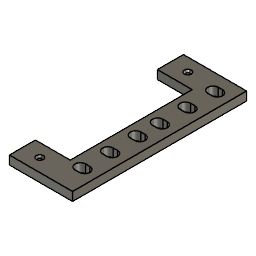
Main (Autodesk Fusion 360 archive; units mm, degrees)
design "Endcaps Right"
Autodesk Fusion 360 part; units mm, degrees
sketch "Sketch1" plane through (0, 0, 0) normal (0, 0, 1) x (1, 0, 0)
  line L0 (0, 0) -> (16.3, 0)
  line L1 (16.3, 0) -> (16.3, 100)
  line L2 (16.3, 100) -> (0, 100)
  line L3 (0, 100) -> (0, 0)
  line L4 (16.3, 100) -> (36.3, 100)
  line L5 (36.3, 100) -> (36.3, 85)
  line L6 (36.3, 85) -> (16.3, 85)
  line L7 (16.3, 85) -> (16.3, 100)
  line L8 (16.3, 0) -> (36.3, 0)
  line L9 (36.3, 0) -> (36.3, 15)
  line L10 (36.3, 15) -> (16.3, 15)
  line L11 (16.3, 15) -> (16.3, 0)
  line L12 (7.5, 87.65) -> (10, 87.65)
  arc A0 (10, 87.65) -> (10, 93.65) centre (10, 90.65) ccw
  line L13 (10, 93.65) -> (7.5, 93.65)
  arc A1 (7.5, 93.65) -> (7.5, 87.65) centre (7.5, 90.65) ccw
  line L14 (7.5, 90.65) -> (10, 90.65) construction
  arc A2 (10, 71.775) -> (10, 77.775) centre (10, 74.775) ccw
  line L15 (7.5, 71.775) -> (10, 71.775)
  arc A3 (7.5, 77.775) -> (7.5, 71.775) centre (7.5, 74.775) ccw
  line L16 (10, 77.775) -> (7.5, 77.775)
  arc A4 (10, 55.9) -> (10, 61.9) centre (10, 58.9) ccw
  line L17 (7.5, 55.9) -> (10, 55.9)
  arc A5 (7.5, 61.9) -> (7.5, 55.9) centre (7.5, 58.9) ccw
  line L18 (10, 61.9) -> (7.5, 61.9)
  line L19 (7.5, 43.2) -> (10, 43.2)
  arc A6 (7.5, 49.2) -> (7.5, 43.2) centre (7.5, 46.2) ccw
  line L20 (10, 49.2) -> (7.5, 49.2)
  arc A7 (10, 43.2) -> (10, 49.2) centre (10, 46.2) ccw
  line L21 (7.5, 27.325) -> (10, 27.325)
  arc A8 (7.5, 33.325) -> (7.5, 27.325) centre (7.5, 30.325) ccw
  line L22 (10, 33.325) -> (7.5, 33.325)
  arc A9 (10, 27.325) -> (10, 33.325) centre (10, 30.325) ccw
  line L23 (7.5, 11.45) -> (10, 11.45)
  arc A10 (7.5, 17.45) -> (7.5, 11.45) centre (7.5, 14.45) ccw
  line L24 (10, 17.45) -> (7.5, 17.45)
  arc A11 (10, 11.45) -> (10, 17.45) centre (10, 14.45) ccw
  circle A12 centre (26.3, 7.5) radius 1
  circle A13 centre (26.3, 92.5) radius 1
  point P0 (8.75, 90.65)
  dimension "d1" = 16.3
  dimension "d2" = 100
  dimension "d3" = 20
  dimension "d4" = 15
  dimension "d5" = 20
  dimension "d19" = 6
  dimension "d20" = 6
  dimension "d21" = 6
  dimension "d22" = 15.875
  dimension "d23" = 15.875
  dimension "d24" = 6
  dimension "d25" = 6
  dimension "d26" = 15.875
  dimension "d27" = 12.7
  dimension "d28" = 6
  dimension "d29" = 15.875
  dimension "d30" = 6.35
  dimension "d33" = 2
  dimension "d34" = 2
  constraint horizontal L0
  constraint vertical L1
  constraint horizontal L2
  constraint vertical L3
  constraint coincident L0.start L3.end
  constraint horizontal L4
  constraint vertical L5
  constraint horizontal L6
  constraint vertical L7
  constraint horizontal L8
  constraint vertical L9
  constraint horizontal L10
  constraint vertical L11
  constraint tangent L12 A0
  constraint tangent A0 L13
  constraint parallel L12 L13
  constraint tangent L13 A1
  constraint tangent L12 A1
  constraint horizontal L14
  constraint midpoint L14 P0
  constraint tangent A2 L15
  constraint tangent A2 L16
  constraint parallel L15 L16
  constraint tangent A3 L16
  constraint tangent L15 A3
  constraint tangent A4 L17
  constraint tangent A4 L18
  constraint parallel L17 L18
  constraint tangent A5 L18
  constraint tangent L17 A5
  constraint tangent L19 A7
  constraint tangent L20 A7
  constraint parallel L19 L20
  constraint tangent A6 L20
  constraint tangent L19 A6
  constraint tangent L21 A9
  constraint tangent L22 A9
  constraint parallel L21 L22
  constraint tangent A8 L22
  constraint tangent L21 A8
  constraint tangent L23 A11
  constraint tangent L24 A11
  constraint parallel L23 L24
  constraint tangent A10 L24
  constraint tangent L23 A10
  measures "d1" distance of L0.start L0.end
  measures "d2" distance of L0.start L2.end
  measures "d3" distance of L1.end L4.end
  measures "d4" distance of L1.end L6.end
  measures "d5" distance of L0.end L8.end
  measures "d19" diameter of A0
  measures "d20" diameter of A2
  measures "d21" diameter of A4
  measures "d22" distance of L13 L16
  measures "d23" distance of L16 L18
  measures "d24" diameter of A7
  measures "d25" diameter of A9
  measures "d26" distance of L20 L22
  measures "d27" distance of L18 L20
  measures "d28" diameter of A11
  measures "d29" distance of L22 L24
  measures "d30" distance of L2 L13
  measures "d33" diameter of A12
  measures "d34" diameter of A13
extrude "Extrude1" add sketch "Sketch1" along normal blind 5
sketch "Sketch2" plane through (0, 0, 5) normal (0, 0, 1) x (-1, 0, 0)
  arc A0 (-10, -11.45) -> (-10, -17.45) centre (-10, -14.45) ccw
  line L0 (-10, -11.45) -> (-7.5, -11.45)
  arc A1 (-7.5, -17.45) -> (-7.5, -11.45) centre (-7.5, -14.45) ccw
  line L1 (-7.5, -17.45) -> (-10, -17.45)
  line L2 (-7.5, -61.9) -> (-10, -61.9)
  arc A2 (-10, -55.9) -> (-10, -61.9) centre (-10, -58.9) ccw
  line L3 (-10, -55.9) -> (-7.5, -55.9)
  arc A3 (-7.5, -61.9) -> (-7.5, -55.9) centre (-7.5, -58.9) ccw
  arc A4 (-7.5, -93.65) -> (-7.5, -87.65) centre (-7.5, -90.65) ccw
  line L4 (-7.5, -93.65) -> (-10, -93.65)
  arc A5 (-10, -87.65) -> (-10, -93.65) centre (-10, -90.65) ccw
  line L5 (-10, -87.65) -> (-7.5, -87.65)
  line L6 (-7.5, -77.775) -> (-10, -77.775)
  arc A6 (-10, -71.775) -> (-10, -77.775) centre (-10, -74.775) ccw
  line L7 (-10, -71.775) -> (-7.5, -71.775)
  arc A7 (-7.5, -77.775) -> (-7.5, -71.775) centre (-7.5, -74.775) ccw
  arc A8 (-10, -43.2) -> (-10, -49.2) centre (-10, -46.2) ccw
  line L8 (-10, -43.2) -> (-7.5, -43.2)
  arc A9 (-7.5, -49.2) -> (-7.5, -43.2) centre (-7.5, -46.2) ccw
  line L9 (-7.5, -49.2) -> (-10, -49.2)
  circle A10 centre (-26.3, -7.5) radius 1
  arc A11 (-10, -27.325) -> (-10, -33.325) centre (-10, -30.325) ccw
  line L10 (-10, -27.325) -> (-7.5, -27.325)
  arc A12 (-7.5, -33.325) -> (-7.5, -27.325) centre (-7.5, -30.325) ccw
  line L11 (-7.5, -33.325) -> (-10, -33.325)
  circle A13 centre (-26.3, -92.5) radius 1
  line L12 (-36.3, -100) -> (0, -100)
  line L13 (0, -100) -> (0, 0)
  line L14 (0, 0) -> (-36.3, 0)
  line L15 (-36.3, 0) -> (-36.3, -15)
  line L16 (-36.3, -15) -> (-16.3, -15)
  line L17 (-16.3, -15) -> (-16.3, -85)
  line L18 (-16.3, -85) -> (-36.3, -85)
  line L19 (-36.3, -85) -> (-36.3, -100)
  circle A14 centre (-26.3, -7.5) radius 2
  circle A15 centre (-26.3, -92.5) radius 2
  dimension "d35" = 4
  dimension "d36" = 4
  constraint concentric A10 A14
  constraint concentric A13 A15
  measures "d35" diameter of A14
  measures "d36" diameter of A15
extrude "Extrude2" cut sketch "Sketch2" along normal blind 4.5 draft -45 from surface at -5 contours A10 | A13 | A14 | A15
move_body "Move1" bodies 1 to x (-1, 0, 0) y (0, 1, 0) z (0, 0, -1) at (36.7067, 0, 10)
move_body "Move2" bodies 1 to x (1, 0, 0) y (0, 1, 0) z (0, 0, 1) at (-0.4067, 0, -5)

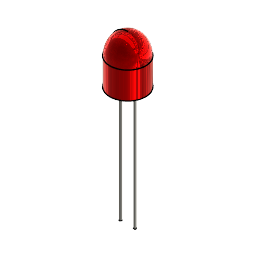
design "LED"
Autodesk Fusion 360 part; units mm, degrees
sketch "Sketch1" plane through (0, 0, 0) normal (0, 0, 1) x (1, 0, 0)
  circle A0 centre (0, 0) radius 1.5
  constraint coincident A0.centre origin
extrude "Extrude1" add sketch "Sketch1" along normal blind 4
fillet "Fillet1" offset 1.49 second offset 1.75 1 edges at (-1.3985, -0.5424, 4) measured on face at (-0.4452, -0.0508, 4)
sketch "Sketch2" plane through (0, 0, 0) normal (0, 0, -1) x (1, 0, 0)
  circle A0 centre (0, 0) radius 1.5
  circle A1 centre (0.6, 0) radius 0.1
  circle A2 centre (-0.6, 0) radius 0.1
extrude "Extrude2" add sketch "Sketch2" along normal blind 10 contours A1 | A2

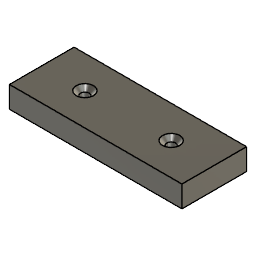
design "Cpnnector"
Autodesk Fusion 360 part; units mm, degrees
sketch "Sketch1" plane through (0, 0, 0) normal (0, 0, 1) x (1, 0, 0)
  line L0 (0, 0) -> (40, 0)
  line L1 (40, 0) -> (40, 15)
  line L2 (40, 15) -> (0, 15)
  line L3 (0, 15) -> (0, 0)
  circle A0 centre (10, 7.5) radius 1
  circle A1 centre (30, 7.5) radius 1
  circle A2 centre (30, 7.5) radius 2
  circle A3 centre (10, 7.5) radius 2
  constraint horizontal L0
  constraint vertical L1
  constraint horizontal L2
  constraint vertical L3
  constraint coincident L0.start L3.end
  constraint concentric A1 A2
  constraint concentric A0 A3
extrude "Extrude1" add sketch "Sketch1" along normal blind 5 contours L0 L1 L2 L3 | A2 | A3
extrude "Extrude2" cut sketch "Sketch1" against normal blind 1 draft -45 from surface at 5 contours A0 | A1 | A2 | A3

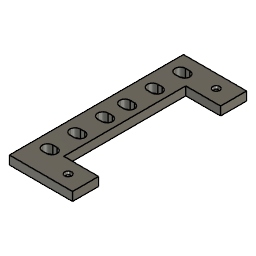
design "Endcaps Left"
Autodesk Fusion 360 part; units mm, degrees
sketch "Sketch1" plane through (0, 0, 0) normal (0, 0, 1) x (1, 0, 0)
  line L0 (0, 0) -> (16.3, 0)
  line L1 (16.3, 0) -> (16.3, 100)
  line L2 (16.3, 100) -> (0, 100)
  line L3 (0, 100) -> (0, 0)
  line L4 (16.3, 100) -> (36.3, 100)
  line L5 (36.3, 100) -> (36.3, 85)
  line L6 (36.3, 85) -> (16.3, 85)
  line L7 (16.3, 85) -> (16.3, 100)
  line L8 (16.3, 0) -> (36.3, 0)
  line L9 (36.3, 0) -> (36.3, 15)
  line L10 (36.3, 15) -> (16.3, 15)
  line L11 (16.3, 15) -> (16.3, 0)
  line L12 (7.5, 87.65) -> (10, 87.65)
  arc A0 (10, 87.65) -> (10, 93.65) centre (10, 90.65) ccw
  line L13 (10, 93.65) -> (7.5, 93.65)
  arc A1 (7.5, 93.65) -> (7.5, 87.65) centre (7.5, 90.65) ccw
  line L14 (7.5, 90.65) -> (10, 90.65) construction
  arc A2 (10, 71.775) -> (10, 77.775) centre (10, 74.775) ccw
  line L15 (7.5, 71.775) -> (10, 71.775)
  arc A3 (7.5, 77.775) -> (7.5, 71.775) centre (7.5, 74.775) ccw
  line L16 (10, 77.775) -> (7.5, 77.775)
  arc A4 (10, 55.9) -> (10, 61.9) centre (10, 58.9) ccw
  line L17 (7.5, 55.9) -> (10, 55.9)
  arc A5 (7.5, 61.9) -> (7.5, 55.9) centre (7.5, 58.9) ccw
  line L18 (10, 61.9) -> (7.5, 61.9)
  line L19 (7.5, 43.2) -> (10, 43.2)
  arc A6 (7.5, 49.2) -> (7.5, 43.2) centre (7.5, 46.2) ccw
  line L20 (10, 49.2) -> (7.5, 49.2)
  arc A7 (10, 43.2) -> (10, 49.2) centre (10, 46.2) ccw
  line L21 (7.5, 27.325) -> (10, 27.325)
  arc A8 (7.5, 33.325) -> (7.5, 27.325) centre (7.5, 30.325) ccw
  line L22 (10, 33.325) -> (7.5, 33.325)
  arc A9 (10, 27.325) -> (10, 33.325) centre (10, 30.325) ccw
  line L23 (7.5, 11.45) -> (10, 11.45)
  arc A10 (7.5, 17.45) -> (7.5, 11.45) centre (7.5, 14.45) ccw
  line L24 (10, 17.45) -> (7.5, 17.45)
  arc A11 (10, 11.45) -> (10, 17.45) centre (10, 14.45) ccw
  circle A12 centre (26.3, 7.5) radius 1
  circle A13 centre (26.3, 92.5) radius 1
  point P0 (8.75, 90.65)
  dimension "d1" = 16.3
  dimension "d2" = 100
  dimension "d3" = 20
  dimension "d4" = 15
  dimension "d5" = 20
  dimension "d19" = 6
  dimension "d20" = 6
  dimension "d21" = 6
  dimension "d22" = 15.875
  dimension "d23" = 15.875
  dimension "d24" = 6
  dimension "d25" = 6
  dimension "d26" = 15.875
  dimension "d27" = 12.7
  dimension "d28" = 6
  dimension "d29" = 15.875
  dimension "d30" = 6.35
  dimension "d33" = 2
  dimension "d34" = 2
  constraint horizontal L0
  constraint vertical L1
  constraint horizontal L2
  constraint vertical L3
  constraint coincident L0.start L3.end
  constraint horizontal L4
  constraint vertical L5
  constraint horizontal L6
  constraint vertical L7
  constraint horizontal L8
  constraint vertical L9
  constraint horizontal L10
  constraint vertical L11
  constraint tangent L12 A0
  constraint tangent A0 L13
  constraint parallel L12 L13
  constraint tangent L13 A1
  constraint tangent L12 A1
  constraint horizontal L14
  constraint midpoint L14 P0
  constraint tangent A2 L15
  constraint tangent A2 L16
  constraint parallel L15 L16
  constraint tangent A3 L16
  constraint tangent L15 A3
  constraint tangent A4 L17
  constraint tangent A4 L18
  constraint parallel L17 L18
  constraint tangent A5 L18
  constraint tangent L17 A5
  constraint tangent L19 A7
  constraint tangent L20 A7
  constraint parallel L19 L20
  constraint tangent A6 L20
  constraint tangent L19 A6
  constraint tangent L21 A9
  constraint tangent L22 A9
  constraint parallel L21 L22
  constraint tangent A8 L22
  constraint tangent L21 A8
  constraint tangent L23 A11
  constraint tangent L24 A11
  constraint parallel L23 L24
  constraint tangent A10 L24
  constraint tangent L23 A10
  measures "d1" distance of L0.start L0.end
  measures "d2" distance of L0.start L2.end
  measures "d3" distance of L1.end L4.end
  measures "d4" distance of L1.end L6.end
  measures "d5" distance of L0.end L8.end
  measures "d19" diameter of A0
  measures "d20" diameter of A2
  measures "d21" diameter of A4
  measures "d22" distance of L13 L16
  measures "d23" distance of L16 L18
  measures "d24" diameter of A7
  measures "d25" diameter of A9
  measures "d26" distance of L20 L22
  measures "d27" distance of L18 L20
  measures "d28" diameter of A11
  measures "d29" distance of L22 L24
  measures "d30" distance of L2 L13
  measures "d33" diameter of A12
  measures "d34" diameter of A13
extrude "Extrude1" add sketch "Sketch1" along normal blind 5
sketch "Sketch2" plane through (0, 0, 5) normal (0, 0, 1) x (-1, 0, 0)
  arc A0 (-10, -11.45) -> (-10, -17.45) centre (-10, -14.45) ccw
  line L0 (-10, -11.45) -> (-7.5, -11.45)
  arc A1 (-7.5, -17.45) -> (-7.5, -11.45) centre (-7.5, -14.45) ccw
  line L1 (-7.5, -17.45) -> (-10, -17.45)
  line L2 (-7.5, -61.9) -> (-10, -61.9)
  arc A2 (-10, -55.9) -> (-10, -61.9) centre (-10, -58.9) ccw
  line L3 (-10, -55.9) -> (-7.5, -55.9)
  arc A3 (-7.5, -61.9) -> (-7.5, -55.9) centre (-7.5, -58.9) ccw
  arc A4 (-7.5, -93.65) -> (-7.5, -87.65) centre (-7.5, -90.65) ccw
  line L4 (-7.5, -93.65) -> (-10, -93.65)
  arc A5 (-10, -87.65) -> (-10, -93.65) centre (-10, -90.65) ccw
  line L5 (-10, -87.65) -> (-7.5, -87.65)
  line L6 (-7.5, -77.775) -> (-10, -77.775)
  arc A6 (-10, -71.775) -> (-10, -77.775) centre (-10, -74.775) ccw
  line L7 (-10, -71.775) -> (-7.5, -71.775)
  arc A7 (-7.5, -77.775) -> (-7.5, -71.775) centre (-7.5, -74.775) ccw
  arc A8 (-10, -43.2) -> (-10, -49.2) centre (-10, -46.2) ccw
  line L8 (-10, -43.2) -> (-7.5, -43.2)
  arc A9 (-7.5, -49.2) -> (-7.5, -43.2) centre (-7.5, -46.2) ccw
  line L9 (-7.5, -49.2) -> (-10, -49.2)
  circle A10 centre (-26.3, -7.5) radius 1
  arc A11 (-10, -27.325) -> (-10, -33.325) centre (-10, -30.325) ccw
  line L10 (-10, -27.325) -> (-7.5, -27.325)
  arc A12 (-7.5, -33.325) -> (-7.5, -27.325) centre (-7.5, -30.325) ccw
  line L11 (-7.5, -33.325) -> (-10, -33.325)
  circle A13 centre (-26.3, -92.5) radius 1
  line L12 (-36.3, -100) -> (0, -100)
  line L13 (0, -100) -> (0, 0)
  line L14 (0, 0) -> (-36.3, 0)
  line L15 (-36.3, 0) -> (-36.3, -15)
  line L16 (-36.3, -15) -> (-16.3, -15)
  line L17 (-16.3, -15) -> (-16.3, -85)
  line L18 (-16.3, -85) -> (-36.3, -85)
  line L19 (-36.3, -85) -> (-36.3, -100)
  circle A14 centre (-26.3, -7.5) radius 2
  circle A15 centre (-26.3, -92.5) radius 2
  dimension "d35" = 4
  dimension "d36" = 4
  constraint concentric A10 A14
  constraint concentric A13 A15
  measures "d35" diameter of A14
  measures "d36" diameter of A15
extrude "Extrude2" cut sketch "Sketch2" against normal blind 4.5 draft -45 contours A10 | A13 | A14 | A15
